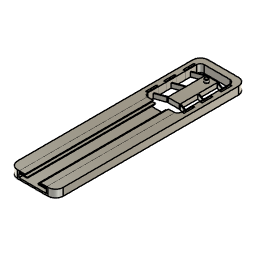
Bistable Blade V3_ (Autodesk Fusion 360 design; units mm, degrees)
Autodesk Fusion 360 part; units mm, degrees
other "Base Mesh Feature1"
sketch "Sketch2" plane through (0, 0, 0) normal (0, 0, 1) x (1, 0, 0)
  line L0 (-15, 72.5) -> (15, 72.5)
  line L1 (15, 72.5) -> (15, -52.5)
  line L2 (15, -52.5) -> (-15, -52.5)
  line L3 (-15, -52.5) -> (-15, 72.5)
  line L4 (-12.5, 41.25) -> (-11.5, 41.25)
  line L5 (-11.5, 41.25) -> (-11.5, 34.2)
  line L6 (-11.5, 34.2) -> (-12.5, 34.2)
  line L7 (-12.5, 34.2) -> (-12.5, 41.25)
  line L8 (-11.5, 46.06) -> (-12.5, 46.06)
  line L9 (-12.5, 53.11) -> (-11.5, 53.11)
  line L10 (-12.5, 46.06) -> (-12.5, 53.11)
  line L11 (-11.5, 53.11) -> (-11.5, 46.06)
  line L12 (-12.5, 65.71) -> (-11.5, 65.71)
  line L13 (-12.5, 58.66) -> (-12.5, 65.71)
  line L14 (-11.5, 58.66) -> (-12.5, 58.66)
  line L15 (-11.5, 65.71) -> (-11.5, 58.66)
  line L16 (12.5, 41.25) -> (12.5, 34.2)
  line L17 (11.5, 53.11) -> (12.5, 53.11)
  line L18 (11.5, 41.25) -> (12.5, 41.25)
  line L19 (12.5, 53.11) -> (12.5, 46.06)
  line L20 (11.5, 34.2) -> (11.5, 41.25)
  line L21 (12.5, 34.2) -> (11.5, 34.2)
  line L22 (11.5, 65.71) -> (12.5, 65.71)
  line L23 (11.5, 46.06) -> (11.5, 53.11)
  line L24 (12.5, 58.66) -> (11.5, 58.66)
  line L25 (12.5, 46.06) -> (11.5, 46.06)
  line L26 (12.5, 65.71) -> (12.5, 58.66)
  line L27 (11.5, 58.66) -> (11.5, 65.71)
  line L28 (-11, 68.5) -> (10.9875, 68.5)
  line L29 (10.9875, 68.5) -> (10.9875, 31.524)
  line L30 (10.9875, 31.524) -> (-11, 31.524)
  line L31 (-11, 31.524) -> (-11, 68.5)
  dimension "d1" = 30
  dimension "d2" = 125
  constraint horizontal L0
  constraint vertical L1
  constraint horizontal L2
  constraint vertical L3
  constraint horizontal L4
  constraint vertical L5
  constraint horizontal L6
  constraint vertical L7
  constraint horizontal L9
  constraint vertical L11
  constraint horizontal L8
  constraint vertical L10
  constraint horizontal L12
  constraint vertical L15
  constraint horizontal L14
  constraint vertical L13
  constraint horizontal L18
  constraint vertical L16
  constraint horizontal L21
  constraint vertical L20
  constraint horizontal L17
  constraint vertical L19
  constraint horizontal L25
  constraint vertical L23
  constraint horizontal L22
  constraint vertical L26
  constraint horizontal L24
  constraint vertical L27
  constraint horizontal L28
  constraint vertical L29
  constraint horizontal L30
  constraint vertical L31
  measures "d1" distance of L0.start L0.end
  measures "d2" distance of L0.start L2.end
extrude "Extrude1" add sketch "Sketch2" along normal blind 5
sketch "Sketch3" plane through (0, 0, 0) normal (0, 0, 1) x (1, 0, 0)
  line L0 (-4, 40) -> (4, 40)
  line L1 (4, 65) -> (-4, 65)
  line L2 (-4, 40) -> (-11, 37.5)
  line L3 (-11, 37.5) -> (-11, 37.985)
  line L4 (-11, 37.985) -> (-4, 40.53)
  line L5 (-4, 52.3625) -> (-11, 49.815)
  line L6 (-11, 49.815) -> (-11, 49.2825)
  line L7 (-11, 49.2825) -> (-4, 51.83)
  line L8 (-4, 65) -> (-11, 62.4525)
  line L9 (-11, 61.92) -> (-4, 64.47)
  line L10 (-11, 62.4525) -> (-11, 61.92)
  line L11 (0, 38.5) -> (0, 36)
  line L12 (11, 61.92) -> (4, 64.47)
  line L13 (4, 40) -> (11, 37.5)
  line L14 (4, 52.3625) -> (11, 49.815)
  line L15 (11, 37.985) -> (4, 40.53)
  line L16 (4, 65) -> (11, 62.4525)
  line L17 (11, 62.4525) -> (11, 61.92)
  line L18 (11, 49.815) -> (11, 49.2825)
  line L19 (11, 49.2825) -> (4, 51.83)
  line L20 (11, 37.5) -> (11, 37.985)
  line L21 (-4, 64.47) -> (-4, 52.3625)
  line L22 (-4, 51.83) -> (-4, 40.53)
  line L23 (4, 40.53) -> (4, 51.83)
  line L24 (4, 52.3625) -> (4, 64.47)
  dimension "d5" = 8
  constraint horizontal L0
  constraint vertical L23
  constraint horizontal L1
  constraint vertical L21
  constraint perpendicular L0 L3
  constraint coincident L4.end L21
  constraint parallel L6 L21
  constraint coincident L7.end L21
  constraint parallel L5 L7
  constraint parallel L5 L8
  constraint parallel L10 L21
  constraint vertical L11
  constraint symmetric L0.start L11 L0.end
  constraint symmetric L1.end L11 L1.start
  constraint symmetric L2.end L11 L13.end
  constraint symmetric L3.end L11 L15.start
  constraint symmetric L4.end L11 L15.end
  constraint symmetric L5.start L11 L14.start
  constraint symmetric L5.end L11 L14.end
  constraint symmetric L6.end L11 L18.end
  constraint symmetric L7.end L11 L19.end
  constraint symmetric L8.end L11 L16.end
  constraint symmetric L9.start L11 L12.start
  constraint symmetric L9.end L11 L12.end
  constraint collinear L21 L22
  constraint collinear L23 L24
  measures "d5" distance of L0.start L0.end
extrude "Extrude2" add sketch "Sketch3" along normal blind 3
fillet "Fillet1" radius 2 2 edges at (-4, 65, 1.5) (4, 65, 1.5)
fillet "Fillet2" radius 2 2 edges at (-4, 40, 1.5) (4, 40, 1.5)
sketch "Sketch4" plane through (0, -52.5, 0) normal (0, -1, 0) x (1, 0, 0)
  line L0 (-15, 0) -> (15, 0)
  line L1 (15, 0) -> (15, 5)
  line L2 (15, 5) -> (-15, 5)
  line L3 (-15, 5) -> (-15, 0)
  line L4 (0, 5) -> (9, 5)
  line L5 (9, 1) -> (-9, 1)
  line L6 (-9, 5) -> (0, 5)
  line L7 (5, 5) -> (5, 4.5)
  line L8 (-5, 4.5) -> (-5, 5)
  line L9 (-9, 4) -> (-3.5, 4)
  line L10 (-3.5, 4) -> (-3.5, 3.5)
  line L11 (-3.5, 3.5) -> (-9, 3.5)
  line L12 (9, 4) -> (3.5, 4)
  line L13 (3.5, 4) -> (3.5, 3.5)
  line L14 (3.5, 3.5) -> (9, 3.5)
  line L15 (-9, 1) -> (-9, 3.5)
  line L16 (-9, 4) -> (-9, 4.5)
  line L17 (-9, 4.5) -> (-5, 4.5)
  line L18 (5, 4.5) -> (9, 4.5)
  line L19 (9, 3.5) -> (9, 1)
  line L20 (9, 4) -> (9, 4.5)
  constraint midpoint L2 L4.start
  constraint coincident L2 L4.end
  constraint coincident L2 L6.start
  constraint perpendicular L2 L15
  constraint coincident L16.end L15
  constraint perpendicular L15 L17
  constraint coincident L7.end L17
  constraint coincident L4 L7.start
  constraint perpendicular L7 L17
  constraint coincident L6 L8.end
  constraint coincident L9.start L15
  constraint perpendicular L9 L15
  constraint perpendicular L9 L10
  constraint perpendicular L11 L15
  constraint perpendicular L12 L13
  constraint collinear L15 L16
  constraint collinear L17 L18
  constraint perpendicular L12 L20
extrude "Extrude3" cut sketch "Sketch4" against normal blind 85 contours L2 L4 L5 L6 L7 L8 L9 L10 L11 L12 L13 L14 L15 L16 L17 L18 L19 L20
fillet "Fillet3" radius 5 4 edges at (15, -52.5, 2.5) (-15, -52.5, 2.5) (15, 72.5, 2.5) (-15, 72.5, 2.5)
fillet "Fillet4" radius 2.5 4 edges at (-11, 68.5, 2.5) (10.9875, 68.5, 2.5) (-11, 31.524, 2.5) (10.9875, 31.524, 2.5)
sketch "Sketch5" plane through (0, 0, 3) normal (0, 0, 1) x (-1, 0, 0)
  arc A0 (-4.3314, -64.8794) -> (-3.6474, -65) centre (-3.6474, -63) ccw
  line L0 (-3.6474, -65) -> (3.6474, -65)
  arc A1 (3.6474, -65) -> (4.3314, -64.8794) centre (3.6474, -63) ccw
  line L1 (4.3314, -64.8794) -> (11, -62.4525)
  line L2 (11, -62.4525) -> (11, -61.92)
  line L3 (11, -61.92) -> (4, -64.47)
  line L4 (4, -64.47) -> (4, -52.3625)
  line L5 (4, -52.3625) -> (11, -49.815)
  line L6 (11, -49.815) -> (11, -49.2825)
  line L7 (11, -49.2825) -> (4, -51.83)
  line L8 (4, -51.83) -> (4, -40.53)
  line L9 (4, -40.53) -> (11, -37.985)
  line L10 (11, -37.985) -> (11, -37.5)
  line L11 (11, -37.5) -> (4.3262, -39.8835)
  arc A2 (3.6536, -40) -> (4.3262, -39.8835) centre (3.6536, -38) ccw
  line L12 (3.6536, -40) -> (-3.6536, -40)
  arc A3 (-4.3262, -39.8835) -> (-3.6536, -40) centre (-3.6536, -38) ccw
  line L13 (-4.3262, -39.8835) -> (-10.9875, -37.5045)
  line L14 (-10.9875, -37.5045) -> (-10.9875, -37.9895)
  line L15 (-10.9875, -37.9895) -> (-4, -40.53)
  line L16 (-4, -40.53) -> (-4, -51.83)
  line L17 (-4, -51.83) -> (-10.9875, -49.2871)
  line L18 (-10.9875, -49.2871) -> (-10.9875, -49.8196)
  line L19 (-10.9875, -49.8196) -> (-4, -52.3625)
  line L20 (-4, -52.3625) -> (-4, -64.47)
  line L21 (-4, -64.47) -> (-10.9875, -61.9246)
  line L22 (-10.9875, -61.9246) -> (-10.9875, -62.457)
  line L23 (-10.9875, -62.457) -> (-4.3314, -64.8794)
  circle A4 centre (0, -62.5) radius 1.25
  dimension "d18" = 2.5
  measures "d18" diameter of A4
extrude "Extrude4" add sketch "Sketch5" along normal blind 2 contours A4
fillet "Fillet5" radius 0.3 1 edges at (1.1654, 62.952, 5)
move_face "MoveFace1" to x (1, 0, 0) y (0, 1, 0) z (0, 0, 1) at (0, -1, 0) 3 faces at (0.5984, 62.6846, 5) (0.5119, 61.3656, 4.7568) (1.1518, 62.9855, 4.1333)
fillet "Fillet6" radius 0.1 1 edges at (1.1654, 61.048, 3)
